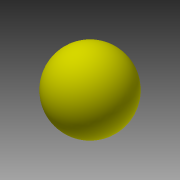
# Autodesk Inventor part: 61816_PART3
Saved by Autodesk Inventor 2014 SP2 (Build 180246200, 246)
## iProperties
Created: 2020-03-09
Part Number: 61816_PART3
Material: Generic
Catalog Web Link: www.cadenas.de
Description: -Deep groove ball bearings
Vendor: SKF
Document SubType Name: Modeling
Designer: psadmin
Manufacturer: SKF
Mass: 0.0898019 g
Surface Area: 0.969783 cm^2
Volume: 0.0898019 cm^3
Density: 1 g/cm^3
Appearance: PSOLRGB-192-192-192
Category: PARTsolutions
Company: SKF
Title: 61816_PART3
Author: Cadenas PARTsolutions
Comments: Deep groove ball bearings
PSOL_IDENT_0: {$CADENAS_DATA\23d-libs\skf\bearings_units_and_housings\ball_bearings\deep_groove_ball_bearings\bb1_
PSOL_IDENT_1: 001_101.prj},188 {VTYP=3D},{NB=61816_PART3},{LINA=61816_PART3},{NN=BB1_001_101_PART3},{NOPRJ=TRUE},{
PSOL_IDENT_2: DATE=19.12.2019 14:34:47},{GEOMDATE=18.12.2019 13:53:11},{VERSION=},{LINEID=6650},{WBVAR=},{WBNUMERI
PSOL_IDENT_3: C=}  {NB=61816_PART3},{LINA=61816_PART3},{KT=DUMMY},{PRODUCTID=1010021816},{DESIGNATION=61816},{DD=8
PSOL_IDENT_4: 0.000},{D=100.000},{B=10.000},{C=0.000},{DD1=86.70},{DD2=0.00},{D1=0.00},{D2=95.70},{D3=0.000},{D4=0
PSOL_IDENT_5: .000},{HH=MIN},{BB=0.000},{FF=0.00},{R0MAX=MIN},{R0=MIN},{R12=1.30},{PITCH=90.00},{DW=5.556},{DDAMIN=
PSOL_IDENT_6: 83.200},{DDAMAX=MIN},{DDBMIN=MIN},{DDBMAX=MIN},{DBMIN=MIN},{DAMAX=96.800},{BBAMIN=MIN},{CAMAX=MIN},{
PSOL_IDENT_7: RAMAX=0.600},{LOAD1=12.700},{LOAD2=11.200},{LOAD3=0.610},{SPEED1=13000},{SPEED2=8000},{KR=0.015},{F0=
PSOL_IDENT_8: 13.300},{Z=27},{II=1},{MASS=0.153},{BEARING=61816},{RING=},{HELP=3.139},{HELP2=2.150},{DD1ALG=43.350
PSOL_IDENT_9: },{YALG=43.350},{PITCH1=90.000},{DW1=5.556},{YALG1=46.861},{HALG1=3.139},{SH=43.350},{CU=0.889},{DES
PSOL_IDENT_10: IGN=dgbb1},{HALG=3.35},{B1=0},{SHIELDHELP=1}
NT: Deep groove ball bearings
NB: 61816_PART3
NBSYN: $DESIGNATION._PART3
LINA: 61816_PART3
SUPPLIER: SKF
ARTICLENO: 61816_PART3
BOMINFO: 61816_PART3
CREATOR: CADENAS GmbH
Autodesk Inventor part; units mm, degrees
ref_plane "YZ Plane" through (0, 0, 0) normal (1, 0, 0) x (0, 1, 0)
ref_plane "XZ Plane" through (0, 0, 0) normal (0, 1, 0) x (-1, 0, 0)
ref_plane "XY Plane" through (0, 0, 0) normal (0, 0, 1) x (1, 0, 0)
sketch "Sketch_6" plane through (0, 0, 0) normal (0, 0, 1) x (1, 0, 0)
  line L0 (7.778, 45) -> (2.222, 45)
  arc A0 (7.778, 45) -> (2.222, 45) centre (5, 45) ccw
  line L1 (7.778, 45) -> (2.222, 45)
  dimension "d0" = 360
  constraints: 4 end point, 2 point on circle, 1 centre point
revolve "Revolution1" add sketch "Sketch_6" angle 360 about axis through (7.778, 45, 0) along (1, 0, 0)
body "Solid1"
